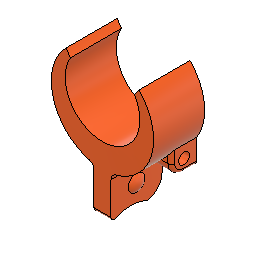
Cushion Holder_v2 (Autodesk Fusion 360 design; units mm, degrees)
Autodesk Fusion 360 part; units mm, degrees
sketch "Sketch1" plane through (0, 0, 0) normal (0, 0, 1) x (1, 0, 0)
  circle A0 centre (0, 0) radius 10.95
  circle A1 centre (0, -3) radius 15
  circle A2 centre (0, 14) radius 12.5
  line L0 (-2.5, -17.7902) -> (-2.5, -30)
  line L1 (-2.5, -30) -> (2.5, -30)
  line L2 (2.5, -30) -> (2.5, -17.7902)
  line L3 (0, 0) -> (0, -30) construction
  line L4 (-12.72, -10.95) -> (12.72, -10.95) construction
  line L5 (-12.72, -17.95) -> (12.72, -17.95)
  line L6 (-12.72, -10.95) -> (-12.72, -17.95)
  line L7 (12.72, -17.95) -> (12.72, -10.95)
  point P0 (0, -30)
  point P1 (0, -10.95)
  point P2 (0, -10.95)
  dimension "d1" = 21.9
  dimension "d2" = 30
  dimension "d3" = 3
  dimension "d4" = 25
  dimension "d5" = 14
  dimension "d21" = 5
  dimension "d22" = 30
  dimension "d25" = 7
  constraint coincident A0.centre L3.start
  constraint vertical A0.centre A1.centre
  constraint vertical A0.centre A2.centre
  constraint vertical L0
  constraint perpendicular L0 L1
  constraint perpendicular L1 L2
  constraint midpoint L1 P0
  constraint vertical A0.centre P0
  constraint coincident A1 L2.end
  constraint coincident A1 L0.start
  constraint coincident P0 L3.end
  constraint coincident L3 P2
  constraint coincident A0 P2
  constraint horizontal L4
  constraint midpoint L4 P2
  constraint coincident P2 P1
  constraint coincident A1 L4.start
  measures "d1" diameter of A0
  measures "d2" diameter of A1
  measures "d3" vertical distance of A0.centre A1.centre
  measures "d4" diameter of A2
  measures "d5" vertical distance of A0.centre A2.centre
  measures "d21" distance of L0.end L1.end
  measures "d22" distance of A0.centre L1
extrude "Extrude1" add sketch "Sketch1" along normal mid plane 15 contours A0 A1 A2 L5 | A1 L5 makes body 1
sketch "Sketch2" plane through (0, 0, 0) normal (1, 0, 0) x (0, 0, -1)
  line L0 (0, 12) -> (0, -18)
  line L1 (0, -10.95) -> (0, -17.95)
  line L2 (0, 0) -> (0, -30)
  point P0 (0, -14.5)
  dimension "d10" = 14.5
  constraint coincident P0 L0
  measures "d10" distance of L2.start P0
extrude "Extrude3" add sketch "Sketch1" along normal mid plane 15 contours A1 L0 L5 | A1 L2 L5 | A1 L0 L1 L2 L5 bodies 1
extrude "Extrude4" add sketch "Sketch1" against normal blind 7.5 contours A1 L0 L5 L6 | A1 L2 L5 L7 bodies 1
hole "Hole2" at (-12.72, -14.45, -3.75) direction (1, 0, 0) diameter 3.2 end through all bodies 1
fillet "Fillet1" radius 3.5 2 edges at (7.61, -17.95, 0) (-7.61, -17.95, 0) on bodies 1
fillet "Fillet2" radius 1 3 edges at (-12.72, -12.7, 0) (-12.72, -16.9249, -1.0251) (-12.72, -17.95, -5.5) on bodies 1
fillet "Fillet3" radius 1 3 edges at (12.72, -17.95, -5.5) (12.72, -16.9249, -1.0251) (12.72, -12.7, 0) on bodies 1
ref_plane "WorkPlane1" through (0, -23.8951, 0) normal (-1, 0, 0) x (0, -1, 0)
sphere "SpherePrimitive1" add diameter 6.973 placed x (0, 0, -1) y (0, -1, 0) z (-1, 0, 0) at (0, -23.8951, 0) bodies 1
fillet "Fillet4" radius 5 1 edges at (0, -30, -7.5) on bodies 1
fillet "Fillet5" radius 2 2 edges at (-2.5, -17.7902, 2.5227) (2.5, -17.7902, 2.5227) on bodies 1
cylinder "CylinderPrimitive1" add diameter 8 height 10 placed x (1, 0, 0) y (0, 1, 0) z (0, 0, 1) at (0, 0, 0) separate body makes body 2 in component "Terminator"
sphere "SpherePrimitive1'" add diameter 8 placed x (1, 0, 0) y (0, 1, 0) z (0, 0, 1) at (0, 0, 10) bodies 2 in component "Terminator"
hole "Hole1" at (0, 0, 0) direction (0, 0, 1) diameter 3.2 depth 10 tip angle 60 bodies 2 in component "Terminator"
chamfer "Chamfer1" distance 1 angle 45 1 edges at (1.4917, 0.5786, 0) on bodies 2 in component "Terminator"
hole "Hole3" at (2.5, -39.9036, 1.664) direction (-1, 0, 0) diameter 22 depth 6 tip angle 118 bodies 1
fillet "Fillet6" radius 1 1 edges at (0, -30, 7.5) on bodies 1
component "Terminator" placed x (1, 0, 0) y (0, 1, 0) z (0, 0, 1) at (0, 0, 0)
equation "d10 = hole_position"
equation "hole_position = 14.5 mm" comment "Pozice otvoru"
named bodies: "Holder", "Terminator"
